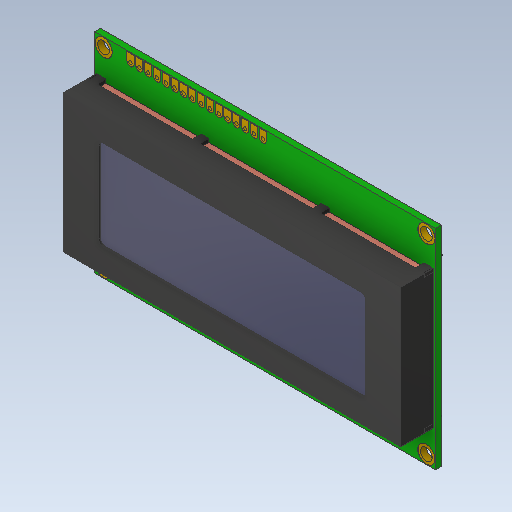
# Autodesk Inventor part: 4x20 LCD
Saved by Autodesk Inventor 2020 (Build 240168000, 168)
## iProperties
Created: 2017-10-08
Part Number: 4x20 LCD
Material: Generic
Document SubType Name: Modeling
Designer: Alex
Density: 1 g/cm^3
Appearance: Default
Author: Alex
Autodesk Inventor part; units mm, degrees
ref_plane "YZ Plane" through (0, 0, 0) normal (1, 0, 0) x (0, 1, 0)
ref_plane "XZ Plane" through (0, 0, 0) normal (0, 1, 0) x (-1, 0, 0)
ref_plane "XY Plane" through (0, 0, 0) normal (0, 0, 1) x (1, 0, 0)
sketch "Sketch1" plane through (0, 0, 0) normal (0, 0, 1) x (1, 0, 0)
  line L0 (49.0474, -30.1117) -> (-49.0474, -30.1117)
  line L1 (-49.0474, -30.1117) -> (-49.0474, 30.1117)
  line L2 (-49.0474, 30.1117) -> (49.0474, 30.1117)
  line L3 (49.0474, 30.1117) -> (49.0474, -30.1117)
  line L4 (49.0474, -30.1117) -> (-49.0474, 30.1117) construction
  line L5 (-49.0474, -30.1117) -> (49.0474, 30.1117) construction
  point P0 (0, 0)
  point P1 (0, 0)
  point P2 (0, 0)
  dimension "d0" = 98.0948
  dimension "d1" = 60.2234
  constraints: 12 end point, 3 midpoint, 2 parallel, 1 coincident, 1 horizontal, 1 perpendicular
  measures "d0" distance of L1.end L2.end
  measures "d1" distance of L0.end L1.end
extrude "Extrusion1" add sketch "Sketch1" along normal mid plane 1.6764
sketch "Sketch2" plane through (0, 0, 0.8382) normal (0, 0, 1) x (1, 0, 0)
  line L0 (46.482, -27.4955) -> (-46.482, -27.4955) construction
  line L1 (-46.482, -27.4955) -> (-46.482, 27.4955) construction
  line L2 (-46.482, 27.4955) -> (46.482, 27.4955) construction
  line L3 (46.482, 27.4955) -> (46.482, -27.4955) construction
  line L4 (46.482, -27.4955) -> (-46.482, 27.4955) construction
  line L5 (-46.482, -27.4955) -> (46.482, 27.4955) construction
  circle A0 centre (-46.482, 27.4955) radius 2.4892
  circle A1 centre (-46.482, -27.4955) radius 2.4892
  circle A2 centre (46.482, 27.4955) radius 2.4892
  circle A3 centre (46.482, -27.4955) radius 2.4892
  point P0 (0, 0)
  dimension "d4" = 92.964
  dimension "d5" = 54.991
  dimension "d6" = 4.9784
  constraints: 12 end point, 4 centre point, 3 coincident, 3 equal radius, 2 midpoint, 2 parallel, 1 horizontal, 1 perpendicular
  measures "d4" distance of L1.end L2.end
  measures "d5" distance of L2.end L0.start
  measures "d6" diameter of A0
extrude "Extrusion2" add sketch "Sketch2" along normal blind 0.0254
mirror "Mirror1" about plane through (0, 0, 0) normal (0, 0, 1) of "Extrusion2"
sketch "Sketch3" plane through (-46.482, 27.4955, 0.8636) normal (0, 0, 1) x (1, 0, 0)
  circle A0 centre (0, 0) radius 2.4892 projected
  circle A1 centre (92.964, 0) radius 2.4892 projected
  circle A2 centre (92.964, -54.991) radius 2.4892 projected
  circle A3 centre (0, -54.991) radius 2.4892 projected
  circle A4 centre (0, 0) radius 2.4892 construction
  line L0 (0, 0) -> (92.964, 0) construction
  line L1 (92.964, 0) -> (92.964, -54.991) construction
  line L2 (92.964, -54.991) -> (0, -54.991) construction
  line L3 (0, -54.991) -> (0, 0) construction
  line L4 (0, 0) -> (92.964, -54.991) construction
  line L5 (92.964, 0) -> (0, -54.991) construction
  point P0 (46.482, -27.4955)
  constraints: 12 end point, 2 parallel, 1 horizontal, 1 perpendicular
hole "Hole1" at (-46.482, 27.4955, 0.8636) at (46.482, 27.4955, 0.8636) at (46.482, -27.4955, 0.8636) at (-46.482, -27.4955, 0.8636) direction (0, 0, -1) diameter 3.429 end through all
sketch "Sketch4" plane through (0, 0, 0.8382) normal (0, 0, 1) x (1, 0, 0)
  line L0 (-39.7764, 27.5971) -> (-39.7764, 29.8577)
  line L1 (-39.7764, 29.8577) -> (-37.6936, 29.8577)
  line L2 (-37.6936, 29.8577) -> (-37.6936, 27.5971)
  arc A0 (-39.7764, 27.5971) -> (-37.6936, 27.5971) centre (-38.735, 27.5971) ccw
  line L3 (-49.0474, 30.1117) -> (-49.0474, -30.1117) projected
  line L4 (49.0474, 30.1117) -> (-49.0474, 30.1117) projected
  line L5 (-37.2364, 27.5971) -> (-37.2364, 29.8577)
  line L6 (-37.2364, 29.8577) -> (-35.1536, 29.8577)
  line L7 (-35.1536, 29.8577) -> (-35.1536, 27.5971)
  arc A1 (-37.2364, 27.5971) -> (-35.1536, 27.5971) centre (-36.195, 27.5971) ccw
  line L8 (-34.6964, 27.5971) -> (-34.6964, 29.8577)
  line L9 (-34.6964, 29.8577) -> (-32.6136, 29.8577)
  line L10 (-32.6136, 29.8577) -> (-32.6136, 27.5971)
  arc A2 (-34.6964, 27.5971) -> (-32.6136, 27.5971) centre (-33.655, 27.5971) ccw
  line L11 (-32.1564, 27.5971) -> (-32.1564, 29.8577)
  line L12 (-32.1564, 29.8577) -> (-30.0736, 29.8577)
  line L13 (-30.0736, 29.8577) -> (-30.0736, 27.5971)
  arc A3 (-32.1564, 27.5971) -> (-30.0736, 27.5971) centre (-31.115, 27.5971) ccw
  line L14 (-29.6164, 27.5971) -> (-29.6164, 29.8577)
  line L15 (-29.6164, 29.8577) -> (-27.5336, 29.8577)
  line L16 (-27.5336, 29.8577) -> (-27.5336, 27.5971)
  arc A4 (-29.6164, 27.5971) -> (-27.5336, 27.5971) centre (-28.575, 27.5971) ccw
  line L17 (-27.0764, 27.5971) -> (-27.0764, 29.8577)
  line L18 (-27.0764, 29.8577) -> (-24.9936, 29.8577)
  line L19 (-24.9936, 29.8577) -> (-24.9936, 27.5971)
  arc A5 (-27.0764, 27.5971) -> (-24.9936, 27.5971) centre (-26.035, 27.5971) ccw
  line L20 (-24.5364, 27.5971) -> (-24.5364, 29.8577)
  line L21 (-24.5364, 29.8577) -> (-22.4536, 29.8577)
  line L22 (-22.4536, 29.8577) -> (-22.4536, 27.5971)
  arc A6 (-24.5364, 27.5971) -> (-22.4536, 27.5971) centre (-23.495, 27.5971) ccw
  line L23 (-21.9964, 27.5971) -> (-21.9964, 29.8577)
  line L24 (-21.9964, 29.8577) -> (-19.9136, 29.8577)
  line L25 (-19.9136, 29.8577) -> (-19.9136, 27.5971)
  arc A7 (-21.9964, 27.5971) -> (-19.9136, 27.5971) centre (-20.955, 27.5971) ccw
  line L26 (-19.4564, 27.5971) -> (-19.4564, 29.8577)
  line L27 (-19.4564, 29.8577) -> (-17.3736, 29.8577)
  line L28 (-17.3736, 29.8577) -> (-17.3736, 27.5971)
  arc A8 (-19.4564, 27.5971) -> (-17.3736, 27.5971) centre (-18.415, 27.5971) ccw
  line L29 (-16.9164, 27.5971) -> (-16.9164, 29.8577)
  line L30 (-16.9164, 29.8577) -> (-14.8336, 29.8577)
  line L31 (-14.8336, 29.8577) -> (-14.8336, 27.5971)
  arc A9 (-16.9164, 27.5971) -> (-14.8336, 27.5971) centre (-15.875, 27.5971) ccw
  line L32 (-14.3764, 27.5971) -> (-14.3764, 29.8577)
  line L33 (-14.3764, 29.8577) -> (-12.2936, 29.8577)
  line L34 (-12.2936, 29.8577) -> (-12.2936, 27.5971)
  arc A10 (-14.3764, 27.5971) -> (-12.2936, 27.5971) centre (-13.335, 27.5971) ccw
  line L35 (-11.8364, 27.5971) -> (-11.8364, 29.8577)
  line L36 (-11.8364, 29.8577) -> (-9.7536, 29.8577)
  line L37 (-9.7536, 29.8577) -> (-9.7536, 27.5971)
  arc A11 (-11.8364, 27.5971) -> (-9.7536, 27.5971) centre (-10.795, 27.5971) ccw
  line L38 (-9.2964, 27.5971) -> (-9.2964, 29.8577)
  line L39 (-9.2964, 29.8577) -> (-7.2136, 29.8577)
  line L40 (-7.2136, 29.8577) -> (-7.2136, 27.5971)
  arc A12 (-9.2964, 27.5971) -> (-7.2136, 27.5971) centre (-8.255, 27.5971) ccw
  line L41 (-6.7564, 27.5971) -> (-6.7564, 29.8577)
  line L42 (-6.7564, 29.8577) -> (-4.6736, 29.8577)
  line L43 (-4.6736, 29.8577) -> (-4.6736, 27.5971)
  arc A13 (-6.7564, 27.5971) -> (-4.6736, 27.5971) centre (-5.715, 27.5971) ccw
  line L44 (-4.2164, 27.5971) -> (-4.2164, 29.8577)
  line L45 (-4.2164, 29.8577) -> (-2.1336, 29.8577)
  line L46 (-2.1336, 29.8577) -> (-2.1336, 27.5971)
  arc A14 (-4.2164, 27.5971) -> (-2.1336, 27.5971) centre (-3.175, 27.5971) ccw
  line L47 (-1.6764, 27.5971) -> (-1.6764, 29.8577)
  line L48 (-1.6764, 29.8577) -> (0.4064, 29.8577)
  line L49 (0.4064, 29.8577) -> (0.4064, 27.5971)
  arc A15 (-1.6764, 27.5971) -> (0.4064, 27.5971) centre (-0.635, 27.5971) ccw
  point P0 (0, 0)
  dimension "d16" = 2.0828
  dimension "d17" = 2.2606
  dimension "d18" = 9.271
  dimension "d19" = 0.254
  dimension "d22" = 2.54
  constraints: 96 end point, 32 point on circle, 16 centre point, 2 perpendicular, 2 tangent, 1 horizontal, 1 vertical, 135 other
  measures "d16" distance between parallel lines of L2 L0
  measures "d17" distance from line of L1 A0.centre
  measures "d18" distance between parallel lines of L3 L0
  measures "d19" distance between parallel lines of L4 L1
  measures "d22" distance of L0.start L5.start
extrude "Extrusion3" add sketch "Sketch4" along normal blind 0.0254
mirror "Mirror2" about plane through (0, 0, 0) normal (0, 0, 1) of "Extrusion3"
sketch "Sketch5" plane through (0, 0, 0.8636) normal (0, 0, 1) x (1, 0, 0)
  line L0 (-4.2164, 29.8577) -> (-2.1336, 29.8577) projected
  line L1 (-2.1336, 29.8577) -> (-2.1336, 27.5971) projected
  arc A0 (-4.2164, 27.5971) -> (-2.1336, 27.5971) centre (-3.175, 27.5971) ccw projected
  line L2 (-4.2164, 27.5971) -> (-4.2164, 29.8577) projected
  line L3 (-9.2964, 29.8577) -> (-7.2136, 29.8577) projected
  line L4 (-7.2136, 29.8577) -> (-7.2136, 27.5971) projected
  arc A1 (-9.2964, 27.5971) -> (-7.2136, 27.5971) centre (-8.255, 27.5971) ccw projected
  line L5 (-9.2964, 27.5971) -> (-9.2964, 29.8577) projected
  line L6 (-14.3764, 29.8577) -> (-12.2936, 29.8577) projected
  line L7 (-12.2936, 29.8577) -> (-12.2936, 27.5971) projected
  arc A2 (-14.3764, 27.5971) -> (-12.2936, 27.5971) centre (-13.335, 27.5971) ccw projected
  line L8 (-14.3764, 27.5971) -> (-14.3764, 29.8577) projected
  line L9 (-19.4564, 29.8577) -> (-17.3736, 29.8577) projected
  line L10 (-17.3736, 29.8577) -> (-17.3736, 27.5971) projected
  arc A3 (-19.4564, 27.5971) -> (-17.3736, 27.5971) centre (-18.415, 27.5971) ccw projected
  line L11 (-19.4564, 27.5971) -> (-19.4564, 29.8577) projected
  line L12 (-24.5364, 29.8577) -> (-22.4536, 29.8577) projected
  line L13 (-22.4536, 29.8577) -> (-22.4536, 27.5971) projected
  arc A4 (-24.5364, 27.5971) -> (-22.4536, 27.5971) centre (-23.495, 27.5971) ccw projected
  line L14 (-24.5364, 27.5971) -> (-24.5364, 29.8577) projected
  line L15 (-29.6164, 29.8577) -> (-27.5336, 29.8577) projected
  line L16 (-27.5336, 29.8577) -> (-27.5336, 27.5971) projected
  arc A5 (-29.6164, 27.5971) -> (-27.5336, 27.5971) centre (-28.575, 27.5971) ccw projected
  line L17 (-29.6164, 27.5971) -> (-29.6164, 29.8577) projected
  line L18 (-34.6964, 29.8577) -> (-32.6136, 29.8577) projected
  line L19 (-32.6136, 29.8577) -> (-32.6136, 27.5971) projected
  arc A6 (-34.6964, 27.5971) -> (-32.6136, 27.5971) centre (-33.655, 27.5971) ccw projected
  line L20 (-34.6964, 27.5971) -> (-34.6964, 29.8577) projected
  line L21 (-39.7764, 29.8577) -> (-37.6936, 29.8577) projected
  line L22 (-37.6936, 29.8577) -> (-37.6936, 27.5971) projected
  arc A7 (-39.7764, 27.5971) -> (-37.6936, 27.5971) centre (-38.735, 27.5971) ccw projected
  line L23 (-39.7764, 27.5971) -> (-39.7764, 29.8577) projected
  line L24 (-37.2364, 29.8577) -> (-35.1536, 29.8577) projected
  line L25 (-35.1536, 29.8577) -> (-35.1536, 27.5971) projected
  arc A8 (-37.2364, 27.5971) -> (-35.1536, 27.5971) centre (-36.195, 27.5971) ccw projected
  line L26 (-37.2364, 27.5971) -> (-37.2364, 29.8577) projected
  line L27 (-32.1564, 29.8577) -> (-30.0736, 29.8577) projected
  line L28 (-30.0736, 29.8577) -> (-30.0736, 27.5971) projected
  arc A9 (-32.1564, 27.5971) -> (-30.0736, 27.5971) centre (-31.115, 27.5971) ccw projected
  line L29 (-32.1564, 27.5971) -> (-32.1564, 29.8577) projected
  line L30 (-27.0764, 29.8577) -> (-24.9936, 29.8577) projected
  line L31 (-24.9936, 29.8577) -> (-24.9936, 27.5971) projected
  arc A10 (-27.0764, 27.5971) -> (-24.9936, 27.5971) centre (-26.035, 27.5971) ccw projected
  line L32 (-27.0764, 27.5971) -> (-27.0764, 29.8577) projected
  line L33 (-21.9964, 29.8577) -> (-19.9136, 29.8577) projected
  line L34 (-19.9136, 29.8577) -> (-19.9136, 27.5971) projected
  arc A11 (-21.9964, 27.5971) -> (-19.9136, 27.5971) centre (-20.955, 27.5971) ccw projected
  line L35 (-21.9964, 27.5971) -> (-21.9964, 29.8577) projected
  line L36 (-16.9164, 29.8577) -> (-14.8336, 29.8577) projected
  line L37 (-14.8336, 29.8577) -> (-14.8336, 27.5971) projected
  arc A12 (-16.9164, 27.5971) -> (-14.8336, 27.5971) centre (-15.875, 27.5971) ccw projected
  line L38 (-16.9164, 27.5971) -> (-16.9164, 29.8577) projected
  line L39 (-11.8364, 29.8577) -> (-9.7536, 29.8577) projected
  line L40 (-9.7536, 29.8577) -> (-9.7536, 27.5971) projected
  arc A13 (-11.8364, 27.5971) -> (-9.7536, 27.5971) centre (-10.795, 27.5971) ccw projected
  line L41 (-11.8364, 27.5971) -> (-11.8364, 29.8577) projected
  line L42 (-6.7564, 29.8577) -> (-4.6736, 29.8577) projected
  line L43 (-4.6736, 29.8577) -> (-4.6736, 27.5971) projected
  arc A14 (-6.7564, 27.5971) -> (-4.6736, 27.5971) centre (-5.715, 27.5971) ccw projected
  line L44 (-6.7564, 27.5971) -> (-6.7564, 29.8577) projected
  line L45 (-1.6764, 29.8577) -> (0.4064, 29.8577) projected
  line L46 (0.4064, 29.8577) -> (0.4064, 27.5971) projected
  arc A15 (-1.6764, 27.5971) -> (0.4064, 27.5971) centre (-0.635, 27.5971) ccw projected
  line L47 (-1.6764, 27.5971) -> (-1.6764, 29.8577) projected
  circle A16 centre (46.482, 27.4955) radius 2.4892 projected
  circle A17 centre (-46.482, 27.4955) radius 2.4892 projected
  circle A18 centre (-46.482, -27.4955) radius 2.4892 projected
  circle A19 centre (46.482, -27.4955) radius 2.4892 projected
  line L48 (-49.0474, -30.1117) -> (49.0474, -30.1117) projected
  line L49 (49.0474, -30.1117) -> (49.0474, 30.1117) projected
  line L50 (49.0474, 30.1117) -> (-49.0474, 30.1117) projected
  line L51 (-49.0474, 30.1117) -> (-49.0474, -30.1117) projected
  point P0 (0, 0)
hole "Hole2" at (-38.735, 27.5971, 0.8636) at (-36.195, 27.5971, 0.8636) at (-33.655, 27.5971, 0.8636) at (-31.115, 27.5971, 0.8636) at (-28.575, 27.5971, 0.8636) at (-26.035, 27.5971, 0.8636) at (-23.495, 27.5971, 0.8636) at (-20.955, 27.5971, 0.8636) at (-18.415, 27.5971, 0.8636) at (-15.875, 27.5971, 0.8636) at (-13.335, 27.5971, 0.8636) at (-10.795, 27.5971, 0.8636) at (-8.255, 27.5971, 0.8636) at (-5.715, 27.5971, 0.8636) at (-3.175, 27.5971, 0.8636) at (-0.635, 27.5971, 0.8636) direction (0, 0, -1) diameter 1.016 end through all
sketch "Sketch6" plane through (0, 0, 0.8382) normal (0, 0, 1) x (1, 0, 0)
  line L0 (48.5394, -19.9009) -> (-48.5394, -19.9009)
  line L1 (-48.5394, -19.9009) -> (-48.5394, 19.9009)
  line L2 (-48.5394, 19.9009) -> (48.5394, 19.9009)
  line L3 (48.5394, 19.9009) -> (48.5394, -19.9009)
  line L4 (48.5394, -19.9009) -> (-48.5394, 19.9009) construction
  line L5 (-48.5394, -19.9009) -> (48.5394, 19.9009) construction
  circle A0 centre (-46.482, 27.4955) radius 1.7145 construction
  point P0 (0, 0)
  dimension "d36" = 97.0788
  dimension "d37" = 39.8018
  dimension "d93" = 7.5946
  constraints: 12 end point, 2 midpoint, 2 parallel, 1 horizontal, 1 perpendicular
  measures "d36" distance of L1.end L2.end
  measures "d37" distance of L0.end L1.end
  measures "d93" distance from line of L2 A0.centre
extrude "Extrusion4" add sketch "Sketch6" along normal blind 9.4488
sketch "Sketch7" plane through (0, 0, 10.287) normal (0, 0, 1) x (1, 0, 0)
  line L0 (37.211, 12.9667) -> (-37.211, 12.9667)
  line L1 (-38.481, 11.6967) -> (-38.481, -11.6967)
  line L2 (-37.211, -12.9667) -> (37.211, -12.9667)
  line L3 (38.481, -11.6967) -> (38.481, 11.6967)
  line L4 (38.481, 12.9667) -> (-38.481, -12.9667) construction
  line L5 (-38.481, 12.9667) -> (38.481, -12.9667) construction
  arc A0 (-37.211, 12.9667) -> (-38.481, 11.6967) centre (-37.211, 11.6967) ccw
  arc A1 (38.481, 11.6967) -> (37.211, 12.9667) centre (37.211, 11.6967) ccw
  arc A2 (37.211, -12.9667) -> (38.481, -11.6967) centre (37.211, -11.6967) ccw
  arc A3 (-38.481, -11.6967) -> (-37.211, -12.9667) centre (-37.211, -11.6967) ccw
  point P0 (0, 0)
  dimension "d40" = 76.962
  dimension "d41" = 25.9334
  dimension "d42" = 1.27
  constraints: 12 end point, 8 point on circle, 8 point on line, 8 tangent, 4 centre point, 3 equal radius, 2 midpoint, 2 parallel, 1 horizontal, 1 perpendicular
  measures "d40" distance of L5.end L4.end
  measures "d41" distance of L5.start L4.end
  measures "d42" radius of A0
extrude "Extrusion5" cut sketch "Sketch7" against normal blind 0.508
sketch "Sketch8" plane through (-48.5394, 19.9009, 0.8382) normal (0, 1, 0) x (1, 0, 0)
  line L0 (0, 0) -> (97.0788, 0) construction
  line L1 (0, 0) -> (0, -9.4488) construction
  line L2 (97.0788, -9.4488) -> (0, -9.4488) construction
  line L3 (97.0788, 0) -> (97.0788, -9.4488) construction
  line L4 (97.0788, 0) -> (0, 0) construction
  line L5 (32.3215, 0) -> (64.7573, 0)
  line L6 (64.7573, 0) -> (64.7573, -2.54)
  line L7 (64.7573, -2.54) -> (32.3215, -2.54)
  line L8 (32.3215, -2.54) -> (32.3215, 0)
  line L9 (66.9481, 0) -> (94.3801, 0)
  line L10 (94.3801, 0) -> (94.3801, -2.54)
  line L11 (94.3801, -2.54) -> (66.9481, -2.54)
  line L12 (66.9481, -2.54) -> (66.9481, 0)
  line L13 (30.1308, 0) -> (2.6987, 0)
  line L14 (2.6987, 0) -> (2.6987, -2.54)
  line L15 (2.6987, -2.54) -> (30.1308, -2.54)
  line L16 (30.1308, -2.54) -> (30.1308, 0)
  line L17 (-0.508, 0) -> (97.5868, 0) projected
  line L18 (0.508, -2.54) -> (2.6987, -2.54) construction
  line L19 (0.3429, 1.7018) -> (0.3429, -0.0254) construction
  line L20 (30.1308, -2.54) -> (32.3215, -2.54) construction
  line L21 (64.7573, -2.54) -> (66.9481, -2.54) construction
  line L22 (96.5708, -2.54) -> (94.3801, -2.54) construction
  line L23 (-0.4318, -0.0254) -> (4.5466, -0.0254) projected
  line L24 (0.127, -0.0254) -> (0.508, -0.0254)
  line L25 (0.508, -0.0254) -> (0.508, -2.54)
  line L26 (0.508, -2.54) -> (0.127, -2.54)
  line L27 (0.127, -2.54) -> (0.127, -0.0254)
  line L28 (96.5708, 0) -> (96.9518, 0)
  line L29 (96.9518, 0) -> (96.9518, -2.54)
  line L30 (96.9518, -2.54) -> (96.5708, -2.54)
  line L31 (96.5708, -2.54) -> (96.5708, 0)
  point P0 (48.5394, 0.8382)
  dimension "d45" = 27.432
  dimension "d46" = 27.432
  dimension "d50" = 32.4358
  dimension "d54" = 2.54
  dimension "d56" = 0.381
  dimension "d57" = 0.127
  dimension "d58" = 0.127
  dimension "d59" = 0.381
  constraints: 48 end point, 11 equal length, 8 perpendicular, 6 horizontal alignment, 5 horizontal, 4 point on line, 3 collinear, 1 other
  measures "d45" distance of L15.end L14.end
  measures "d46" distance of L10.end L11.end
  measures "d50" distance of L6.end L7.end
  measures "d54" distance of L13.end L14.end
  measures "d56" distance between parallel lines of L27 L25
  measures "d57" distance between parallel lines of L1 L27
  measures "d58" distance between parallel lines of L3 L29
  measures "d59" distance of L28.start L28.end
extrude "Extrusion6" cut sketch "Sketch8" against normal blind 1.016
mirror "Mirror3" about plane through (0, 0, 0) normal (0, 1, 0) of "Extrusion6"
sketch "Sketch9" plane through (0, 0, -0.8382) normal (0, 0, -1) x (-1, 0, 0)
  line L0 (-46.3441, 20.7391) -> (-42.7355, 17.1635)
  line L1 (-42.7355, 17.1635) -> (-43.3433, 16.5501)
  line L2 (-43.3433, 16.5501) -> (-46.9519, 20.1256)
  line L3 (-46.9519, 20.1256) -> (-46.3441, 20.7391)
  line L4 (-46.3441, 20.7391) -> (-43.3433, 16.5501) construction
  line L5 (-42.7355, 17.1635) -> (-46.9519, 20.1256) construction
  line L6 (-46.8122, -19.9478) -> (-43.2036, -16.3723)
  line L7 (-43.2036, -16.3723) -> (-42.5958, -16.9857)
  line L8 (-42.5958, -16.9857) -> (-46.2044, -20.5613)
  line L9 (-46.2044, -20.5613) -> (-46.8122, -19.9478)
  line L10 (-46.8122, -19.9478) -> (-42.5958, -16.9857) construction
  line L11 (-43.2036, -16.3723) -> (-46.2044, -20.5613) construction
  line L12 (-39.3887, 34.7813) -> (-34.3087, 34.7813) construction
  line L13 (-34.3087, 34.7813) -> (-34.3087, 33.9177) construction
  line L14 (-34.3087, 33.9177) -> (-39.3887, 33.9177) construction
  line L15 (-39.3887, 33.9177) -> (-39.3887, 34.7813) construction
  line L16 (-49.0474, 30.1117) -> (-49.0474, -30.1117) construction
  line L17 (49.0474, 30.1117) -> (-49.0474, 30.1117) construction
  line L18 (-49.0474, -30.1117) -> (49.0474, -30.1117) construction
  line L19 (-18.5293, 20.1256) -> (-17.9215, 20.7391)
  line L20 (-14.3129, 17.1635) -> (-14.9207, 16.5501)
  line L21 (-17.9215, 20.7391) -> (-14.3129, 17.1635)
  line L22 (-14.3129, 17.1635) -> (-18.5293, 20.1256) construction
  line L23 (-17.9215, 20.7391) -> (-14.9207, 16.5501) construction
  line L24 (-14.9207, 16.5501) -> (-18.5293, 20.1256)
  line L25 (-14.781, -16.3723) -> (-14.1732, -16.9857)
  line L26 (-18.3896, -19.9478) -> (-14.1732, -16.9857) construction
  line L27 (-18.3896, -19.9478) -> (-14.781, -16.3723)
  line L28 (-14.1732, -16.9857) -> (-17.7818, -20.5613)
  line L29 (-14.781, -16.3723) -> (-17.7818, -20.5613) construction
  line L30 (-17.7818, -20.5613) -> (-18.3896, -19.9478)
  line L31 (0, 0) -> (0, -25.1815) construction
  line L32 (46.3441, 20.7391) -> (42.7355, 17.1635)
  line L33 (42.7355, 17.1635) -> (43.3433, 16.5501)
  line L34 (43.3433, 16.5501) -> (46.9519, 20.1256)
  line L35 (46.9519, 20.1256) -> (46.3441, 20.7391)
  line L36 (46.3441, 20.7391) -> (43.3433, 16.5501) construction
  line L37 (42.7355, 17.1635) -> (46.9519, 20.1256) construction
  line L38 (46.8122, -19.9478) -> (43.2036, -16.3723)
  line L39 (43.2036, -16.3723) -> (42.5958, -16.9857)
  line L40 (42.5958, -16.9857) -> (46.2044, -20.5613)
  line L41 (46.2044, -20.5613) -> (46.8122, -19.9478)
  line L42 (46.8122, -19.9478) -> (42.5958, -16.9857) construction
  line L43 (43.2036, -16.3723) -> (46.2044, -20.5613) construction
  line L44 (18.5293, 20.1256) -> (17.9215, 20.7391)
  line L45 (14.3129, 17.1635) -> (14.9207, 16.5501)
  line L46 (17.9215, 20.7391) -> (14.3129, 17.1635)
  line L47 (14.3129, 17.1635) -> (18.5293, 20.1256) construction
  line L48 (17.9215, 20.7391) -> (14.9207, 16.5501) construction
  line L49 (14.9207, 16.5501) -> (18.5293, 20.1256)
  line L50 (14.781, -16.3723) -> (14.1732, -16.9857)
  line L51 (18.3896, -19.9478) -> (14.1732, -16.9857) construction
  line L52 (18.3896, -19.9478) -> (14.781, -16.3723)
  line L53 (14.1732, -16.9857) -> (17.7818, -20.5613)
  line L54 (14.781, -16.3723) -> (17.7818, -20.5613) construction
  line L55 (17.7818, -20.5613) -> (18.3896, -19.9478)
  point P0 (-44.8437, 18.6446)
  point P1 (-44.704, -18.4668)
  point P2 (-16.4211, 18.6446)
  point P3 (-16.2814, -18.4668)
  point P4 (44.8437, 18.6446)
  point P5 (44.704, -18.4668)
  point P6 (16.4211, 18.6446)
  point P7 (16.2814, -18.4668)
  dimension "d60" = 5.08
  dimension "d61" = 0.8636
  dimension "d62" = 2.0955
  dimension "d63" = 9.3726
  dimension "d64" = 4.2164
  dimension "d65" = 2.2352
  dimension "d66" = 9.5504
  dimension "d67" = 4.2164
  dimension "d70" = 28.4226
  constraints: 106 end point, 20 symmetric about line, 16 midpoint, 6 parallel, 4 equal length, 3 perpendicular, 2 horizontal, 1 vertical, 22 other
  measures "d60" distance of L12.start L12.end
  measures "d61" distance of L14.end L12.start
  measures "d62" distance from line of L16 L2.end
  measures "d63" distance from line of L17 L0.start
  measures "d64" horizontal distance of L2.end L0.end
  measures "d65" distance from line of L16 L6.start
  measures "d66" distance from line of L18 L8.end
  measures "d67" horizontal distance of L6.start L7.end
  measures "d70" distance of L0.start L19.end
extrude "Extrusion7" add sketch "Sketch9" along normal blind 2.54
sketch "Sketch10" plane through (0, 0, -0.8382) normal (0, 0, -1) x (-1, 0, 0)
  circle A0 centre (-27.1526, -0.8763) radius 5.0165
  circle A1 centre (-12.7254, 7.6327) radius 5.0165
  circle A2 centre (-4.5974, -8.9789) radius 5.0165
  circle A3 centre (24.2062, -9.3853) radius 5.0165
  circle A4 centre (16.891, 6.8961) radius 5.0165
  line L0 (-49.0474, 30.1117) -> (-49.0474, -30.1117) projected
  line L1 (49.0474, 30.1117) -> (-49.0474, 30.1117) projected
  line L2 (-49.0474, -30.1117) -> (49.0474, -30.1117) projected
  line L3 (49.0474, -30.1117) -> (49.0474, 30.1117) projected
  point P0 (0, 0)
  dimension "d77" = 10.033
  dimension "d78" = 21.8948
  dimension "d79" = 30.988
  dimension "d80" = 36.322
  dimension "d81" = 22.479
  dimension "d82" = 44.45
  dimension "d83" = 21.1328
  dimension "d84" = 23.2156
  dimension "d85" = 32.1564
  dimension "d86" = 24.8412
  dimension "d87" = 20.7264
  constraints: 5 centre point, 4 equal radius
  measures "d77" diameter of A0
  measures "d78" distance from line of L0 A0.centre
  measures "d79" distance from line of L1 A0.centre
  measures "d80" distance from line of L0 A1.centre
  measures "d81" distance from line of L1 A1.centre
  measures "d82" distance from line of L0 A2.centre
  measures "d83" distance from line of L2 A2.centre
  measures "d84" distance from line of L1 A4.centre
  measures "d85" distance from line of L3 A4.centre
  measures "d86" distance from line of L3 A3.centre
  measures "d87" distance from line of L2 A3.centre
extrude "Extrusion8" add sketch "Sketch10" along normal blind 1.3716 contours A0 | A1 | A2 | A3 | A4
fillet "Fillet1" radius 4.826 1 edges at (32.1691, -0.8763, -2.2098)
fillet "Fillet2" radius 4.826 4 edges at (17.7419, 7.6327, -2.2098) (9.6139, -8.9789, -2.2098) (-11.8745, 6.8961, -2.2098) (-19.1897, -9.3853, -2.2098)
equation "\"d46\" = d45"
equation "\"d67\" = d64"
body "Solid1"
